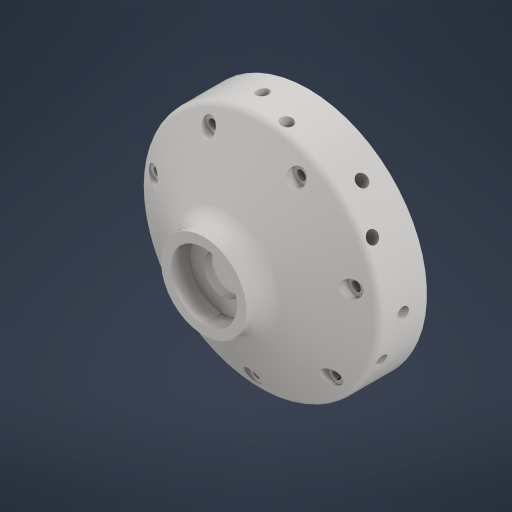
# Autodesk Inventor part: Drum
Saved by Autodesk Inventor 2023 (Build 270158000, 158)
## iProperties
Created: 2025-05-22
Part Number: Drum
Material: Generic
Document SubType Name: Modeling
Designer: ryzen
Density: 1 g/cm^3
Appearance: Default
Author: ryzen
Autodesk Inventor part; units mm, degrees
ref_plane "YZ Plane" through (0, 0, 0) normal (1, 0, 0) x (0, 1, 0)
ref_plane "XZ Plane" through (0, 0, 0) normal (0, 1, 0) x (-1, 0, 0)
ref_plane "XY Plane" through (0, 0, 0) normal (0, 0, 1) x (1, 0, 0)
sketch "Sketch1" plane through (0, 0, 0) normal (1, 0, 0) x (0, 1, 0)
  line L0 (8, 14.9516) -> (8, 11.4516)
  line L1 (8, 11.4516) -> (17.0306, 11.4516)
  line L2 (17.0306, 11.4516) -> (36.0783, 1.9257)
  line L3 (40.5, -5.2294) -> (40.5, -17.0484)
  line L4 (40.5, -17.0484) -> (45, -17.0484)
  line L5 (45, -17.0484) -> (45, -21.0484)
  line L6 (45, -21.0484) -> (50, -21.0484)
  line L7 (50, -21.0484) -> (50, -2.9773)
  line L8 (48.3419, -0.2941) -> (22.4217, 12.6688)
  line L9 (18, 19.8239) -> (18, 22.9516)
  line L10 (18, 22.9516) -> (14, 22.9516)
  line L11 (14, 22.9516) -> (14, 14.9516)
  line L12 (14, 14.9516) -> (8, 14.9516)
  line L13 (0, 31.7516) -> (0, -29.8484) projected
  arc A0 (18, 19.8239) -> (22.4217, 12.6688) centre (26, 19.8239) ccw
  arc A1 (40.5, -5.2294) -> (36.0783, 1.9257) centre (32.5, -5.2294) ccw
  arc A2 (50, -2.9773) -> (48.3419, -0.2941) centre (47, -2.9773) ccw
  point P0 (42.75, -17.0484)
  point P1 (47.5, -21.0484)
  dimension "d4" = 50
  dimension "d5" = 45
  dimension "d6" = 40.5
  dimension "d7" = 4
  dimension "d8" = 32.5
  dimension "d9" = 44
  dimension "d10" = 3.5
  dimension "d11" = 18
  dimension "d12" = 14
  dimension "d13" = 26.57
  dimension "d14" = 8
  dimension "d15" = 3.5
  dimension "d16" = 8
  dimension "d17" = 8
  dimension "d18" = 3
  constraints: 26 end point, 8 perpendicular, 6 point on circle, 6 tangent, 3 centre point, 3 parallel, 2 midpoint, 1 vertical
  measures "d4" distance between parallel lines of L13 L7
  measures "d5" distance between parallel lines of L13 L5
  measures "d6" distance between parallel lines of L13 L3
  measures "d7" distance from line of L6 point (42.75, -17.048)
  measures "d8" distance from line of point (47.5, -21.048) L1
  measures "d9" distance between parallel lines of L6 L10
  measures "d10" distance between parallel lines of L2 L8
  measures "d11" distance between parallel lines of L13 L9
  measures "d12" distance between parallel lines of L13 L11
  measures "d13" angle of L2 L6
  measures "d14" distance between parallel lines of L13 L0
  measures "d15" distance between parallel lines of L1 L12
  measures "d16" radius of A0
  measures "d17" radius of A1
  measures "d18" radius of A2
revolve "Revolution1" add sketch "Sketch1" angle 360 about axis through (0, 0, 0) along (0, 0, -1)
sketch "Sketch2" plane through (0, 0, 0) normal (0, 1, 0) x (-1, 0, 0)
  circle A0 centre (9.21, -11.0484) radius 2.5
  circle A1 centre (-7, -5.0484) radius 2.5
  line L0 (0, 0) -> (0, -61.1407) construction
  line L1 (-50, -21.0484) -> (50, -21.0484) construction
  dimension "d20" = 5
  dimension "d21" = 7
  dimension "d22" = 9.21
  dimension "d23" = 10
  dimension "d24" = 16
  constraints: 2 centre point, 2 end point, 1 equal radius, 1 vertical
  measures "d20" diameter of A0
  measures "d21" distance from line of L0 A1.centre
  measures "d22" distance from line of L0 A0.centre
  measures "d23" distance from line of A0.centre L1
  measures "d24" distance from line of L1 A1.centre
extrude "Extrusion1" cut sketch "Sketch2" along normal blind 55.75
sketch "Sketch3" plane through (0, 0, -17.0484) normal (0, 0, -1) x (-1, 0, 0)
  circle A0 centre (0, 0) radius 40.5 projected
  point P0 (0, -42.75)
  point P1 (0, -40.5)
  dimension "d27" = 2.25
  constraints: 1 vertical alignment, 1 other
  measures "d27" distance of point (0, -42.75) point (0, -40.5)
hole "Hole1" at (0, -42.75, -17.0484) direction (0, 0, 1) diameter 4 end through all
sketch "Sketch4" plane through (0, 0, 0) normal (1, 0, 0) x (0, 1, 0)
  line L0 (-45, -17.0484) -> (45, -17.0484) projected
  line L1 (-42.75, -17.0484) -> (-42.75, 4.5717)
  line L2 (-40.75, 3.5026) -> (-40.75, -17.0484) projected
  line L3 (-40.75, -18.7291) -> (-42.75, -18.7291)
  line L4 (-40.75, 3.5026) -> (-42.75, 3.5026)
  line L5 (-42.75, 0.4516) -> (-39.25, 0.4516)
  line L6 (-39.25, 0.4516) -> (-39.25, 5.4516)
  line L7 (-39.25, 5.4516) -> (-42.75, 5.4516)
  line L8 (-42.75, 0.4516) -> (-42.75, 5.4516)
  point P0 (0, 0)
  dimension "d35" = 2
  dimension "d36" = 5
  dimension "d37" = 3.5
  dimension "d38" = 3.5
  dimension "d39" = 17.5
  constraints: 14 end point, 5 perpendicular, 5 point on line, 1 horizontal
  measures "d35" distance of L3.start L3.end
  measures "d36" distance of L5.end L6.end
  measures "d37" distance of L6.end L7.end
  measures "d38" distance of L5.start L5.end
  measures "d39" distance between parallel lines of L0 L5
revolve "Revolution2" cut sketch "Sketch4" angle 360 about axis through (0, -42.75, -17.0484) along (0, 0, 1) contours L1 L4 L2 L5 | L2 L4 L1 L8 L7 L6 L5
pattern_circular "Circular Pattern1" count 7 over 360 about axis through (0, 0, -10) along (0, 0, 1) of "Hole1", "Revolution2", "Extrusion1"
body "Solid1"
